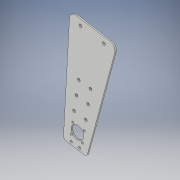
# Autodesk Inventor part: lifterMountMetal
Saved by Autodesk Inventor 2017 (Build 210142000, 142)
## iProperties
Created: 2017-02-04
Part Number: lifterMountMetal
Material: Generic
Document SubType Name: Sheet Metal
Designer: kingb
Density: 1 g/cm^3
Sheet Metal Rule: Default
Appearance: Default
Author: kingb
Autodesk Inventor part; units mm, degrees
ref_plane "YZ Plane" through (0, 0, 0) normal (1, 0, 0) x (0, 1, 0)
ref_plane "XZ Plane" through (0, 0, 0) normal (0, 1, 0) x (-1, 0, 0)
ref_plane "XY Plane" through (0, 0, 0) normal (0, 0, 1) x (1, 0, 0)
ref_plane "Work Plane1" through (187.0611, 458.9587, 0) normal (0, 0, 1) x (0.1591916, 0.9872477, 0)
sketch "Sketch1" plane through (187.0611, 458.9587, 0) normal (0, 0, 1) x (0.1591916, 0.9872477, 0)
  line L0 (5.0953, 0.0423) -> (5.0108, 609.6423)
  line L1 (-36.1797, 0.0366) -> (-36.2642, 609.6366)
  line L2 (-87.0268, 299.6189) -> (-40.0368, 299.6189)
  line L3 (5.0667, 206.0736) -> (-239.4228, 300.8893)
  line L4 (-87.0268, 401.2189) -> (-239.4268, 401.2189)
  line L5 (5.0265, 496.0682) -> (-239.4268, 401.2189)
  circle A0 centre (-207.6768, 350.4189) radius 15.4305 construction
  circle A1 centre (-207.6768, 350.4189) radius 13.0556 construction
  circle A2 centre (-207.6767, 351.037) radius 12.7
  line L6 (5.0466, 351.0648) -> (-194.9767, 351.037)
  line L7 (-220.3767, 351.037) -> (-239.4267, 351.037)
  line L8 (-239.4267, 351.037) -> (-239.4267, 325.637)
  line L9 (-239.4267, 351.037) -> (-239.4267, 376.437)
  line L10 (-239.4267, 325.637) -> (5.0537, 300.2648)
  line L11 (-239.4267, 376.437) -> (5.0396, 401.8648)
  point P0 (-482.8845, 111.6133)
  point P1 (5.0526, 307.6736)
  point P2 (5.0406, 394.4682)
  point P3 (5.0304, 467.7016)
  point P4 (5.0628, 234.4154)
  point P5 (-239.4268, 372.8507)
  dimension "d0" = 101.6
  dimension "d1" = 101.6
  dimension "d2" = 233.2861
  dimension "d30" = 244.4764
  dimension "d35" = 25.4
  dimension "d38" = 25.4
  dimension "d39" = 25.4
  dimension "d40" = 200.0234
  dimension "d41" = 50.8
  dimension "d42" = 50.8
  dimension "d43" = 19.05
  dimension "d44" = 25.4277
  dimension "d45" = 25.3723
  measures "d0" distance of point (5.053, 307.674) L3.start
  measures "d1" distance of point (5.041, 394.468) L5.start
  measures "d2" distance of point (5.03, 467.702) point (5.063, 234.415)
  measures "d30" distance from line of L0 L3.end
  measures "d35" diameter of A2
  measures "d38" distance of L7.end L8.end
  measures "d39" distance of L7.end L9.end
  measures "d40" distance of L6.start L6.end
  measures "d41" distance of L6.start L11.end
  measures "d42" distance of L10.end L6.start
  measures "d43" distance of L7.end L7.start
  measures "d44" vertical distance of L11.end L9.end
  measures "d45" vertical distance of L10.end L8.end
extrude "Plate1" add sketch "Sketch1" along normal blind 3.048 contours L10 L1 L6 L0 | L6 L1 L11 L0 | L10 L8 L7 A2 L6 L1 | L6 A2 L7 L9 L11 L1
sketch "Sketch2" plane through (187.0611, 458.9587, 3.048) normal (0, 0, 1) x (0.1591916, 0.9872477, 0)
  circle A0 centre (-195.4493, 362.9394) radius 2.1463 projected
  circle A1 centre (-220.1972, 362.6464) radius 2.1463 projected
  circle A2 centre (-219.9042, 337.8985) radius 2.1463 projected
  circle A3 centre (-195.1563, 338.1915) radius 2.1463 projected
  point P0 (-482.8845, 111.6133)
extrude "Extrusion1" cut sketch "Sketch2" against normal up to surface (3.048 mm away)
sketch "Sketch3" plane through (187.0611, 458.9587, 3.048) normal (0, 0, 1) x (0.1591916, 0.9872477, 0)
  circle A0 centre (-207.6767, 351.037) radius 12.7 projected
  circle A1 centre (-207.6767, 351.037) radius 13.4937
  point P0 (-482.8845, 111.6133)
  point P1 (-207.6768, 350.4189)
  dimension "d36" = 0.7937
  constraints: 1 centre point
  measures "d36" radial gap between concentric circles of A0 A1
extrude "Extrusion2" cut sketch "Sketch3" against normal up to surface (3.048 mm away)
sketch "Sketch5" plane through (187.0611, 458.9587, 3.048) normal (0, 0, 1) x (0.9872477, -0.1591916, 0)
  line L0 (-401.8648, 5.0396) -> (-300.2648, 5.0537) projected
  line L1 (-300.2648, 5.0537) -> (-401.8648, 5.0396) construction
  line L2 (-319.3169, 5.051) -> (-319.3151, -7.649) construction
  line L3 (-401.8648, 5.0396) -> (-376.437, -239.4267) projected
  line L4 (-319.3151, -7.649) -> (-301.583, -7.649)
  line L5 (-300.2648, 5.0537) -> (-325.637, -239.4267) projected
  circle A0 centre (-376.4648, -7.649) radius 3.175
  circle A1 centre (-325.6648, -7.649) radius 3.175
  line L6 (-319.3151, -7.649) -> (-322.4898, -7.649)
  line L7 (-328.8398, -7.649) -> (-373.2898, -7.649)
  line L8 (-379.6398, -7.649) -> (-400.545, -7.649)
  point P0 (-111.6133, -482.8845)
  point P1 (-351.0648, 5.0466)
  dimension "d47" = 12.7
  dimension "d48" = 12.7025
  dimension "d49" = 6.35
  dimension "d50" = 6.35
  dimension "d51" = 50.8
  dimension "d52" = 50.8
  dimension "d53" = 25.4
  constraints: 10 end point, 4 horizontal, 4 point on circle, 4 point on line, 2 centre point, 1 midpoint, 1 perpendicular
  measures "d47" distance of L2.start L2.end
  measures "d48" distance from line of L0 L4.end
  measures "d49" diameter of A0
  measures "d50" diameter of A1
  measures "d51" distance of A0.centre A1.centre
  measures "d52" distance of L0.end point (-351.065, 5.047)
  measures "d53" horizontal distance of point (-351.065, 5.047) A0.centre
sketch "Sketch6" plane through (187.0611, 458.9587, 0) normal (0, 0, -1) x (-0.9872477, 0.1591916, 0)
  circle A0 centre (337.8985, -219.9042) radius 2.1463
  circle A1 centre (338.1915, -195.1563) radius 2.1463
  circle A2 centre (362.6464, -220.1972) radius 2.1463
  circle A3 centre (362.9394, -195.4493) radius 2.1463
  line L0 (325.637, -239.4267) -> (376.437, -239.4267)
  line L1 (300.2648, 5.0537) -> (325.637, -239.4267)
  line L2 (376.437, -239.4267) -> (401.8648, 5.0396)
  line L3 (401.8648, 5.0396) -> (300.2648, 5.0537)
  circle A4 centre (338.337, -172.7517) radius 2.9337
  circle A5 centre (338.337, -141.0017) radius 2.9337
  circle A6 centre (363.737, -141.0017) radius 2.9337
  circle A7 centre (363.737, -172.7517) radius 2.9337
  circle A8 centre (338.337, -109.2517) radius 2.9337
  circle A9 centre (363.737, -109.2517) radius 2.9337
  point P0 (111.6133, -482.8845)
extrude "Extrusion5" cut sketch "Sketch6" against normal up to next contours A4 | A5 | A6 | A7 | A8 | A9
sketch "Sketch7" plane through (187.0611, 458.9587, 0) normal (0, 0, -1) x (-0.9872477, 0.1591916, 0)
  circle A0 centre (360.3613, -233.0767) radius 2.54 projected
  circle A1 centre (342.275, -233.0767) radius 2.54 projected
  point P0 (111.6133, -482.8845)
extrude "Extrusion6" cut sketch "Sketch7" against normal up to next
extrude "Extrusion7" cut sketch "Sketch5" against normal up to next contours A0 | A1
fillet "Fillet1" radius 12.7 2 edges at (-108.57, 511.7476, 1.524) (-208.8766, 527.9075, 1.524)
fillet "Fillet2" radius 6.35 2 edges at (-222.6902, 282.5108, 1.524) (-172.538, 274.4239, 1.524)
equation "\"BendRadius\" = Thickness"
equation "\"BendReliefWidth\" = Thickness"
equation "\"BendReliefDepth\" = 0.5 * Thickness"
equation "\"CornerReliefSize\" = 4 * Thickness"
equation "\"MinimumRemnant\" = 2 * Thickness"
equation "\"TransitionRadius\" = BendRadius"
equation "\"JacobiRadiusSize\" = BendRadius"
equation "\"GapSize\" = Thickness"
equation "\"d4\" = BendRadius"
equation "\"Thickness\" = 3.048"
body "Solid1"
